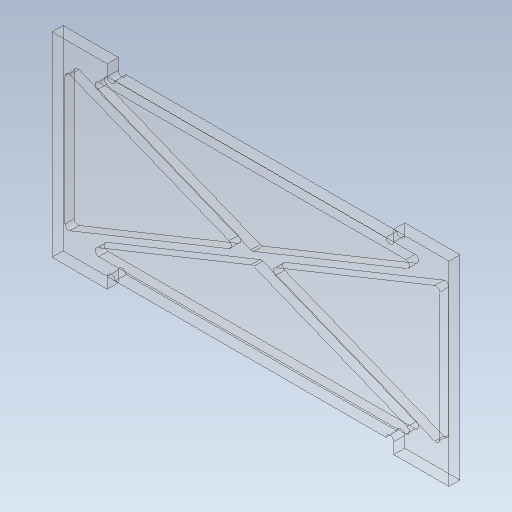
# Autodesk Inventor part: 台形サスバー板
Saved by Autodesk Inventor 2020 (Build 240168000, 168)
## iProperties
Created: 2019-09-18
Part Number: 台形サスバー板
Material: ポリカーボネート、クリア
Document SubType Name: Modeling
Designer: tanjihayato
Density: 1.2 g/cm^3
Appearance: ポリカーボネート - クリア
Mass: 18.8575 g
Surface Area: 114.914 cm^2
Volume: 15.7145 cm^3
Author: tanjihayato
Autodesk Inventor part; units mm, degrees
ref_plane "YZ Plane" through (0, 0, 0) normal (1, 0, 0) x (0, 1, 0)
ref_plane "XZ Plane" through (0, 0, 0) normal (0, 1, 0) x (-1, 0, 0)
ref_plane "XY Plane" through (0, 0, 0) normal (0, 0, 1) x (1, 0, 0)
sketch "スケッチ1" plane through (0, 0, 0) normal (0, 0, 1) x (1, 0, 0)
  circle A0 centre (-35.9404, 22.842) radius 1.5
  circle A1 centre (5.9362, 53.5882) radius 1.5
  circle A2 centre (127.6431, 30.2622) radius 1.5
  line L0 (22.1499, 50.4807) -> (113.9448, 32.8876)
  circle A3 centre (5.9362, 53.5882) radius 4.5
  circle A4 centre (127.6431, 30.2622) radius 4.5
  circle A5 centre (-35.9404, 22.842) radius 3
  line L1 (5.0892, 49.1686) -> (11.145, 48.008)
  line L2 (11.145, 48.008) -> (22.1499, 50.4807)
  line L3 (113.9448, 32.8876) -> (122.4523, 26.6751)
  line L4 (122.4523, 26.6751) -> (126.7961, 25.8426)
  line L5 (4.4419, 57.8328) -> (15.2047, 61.622)
  line L6 (-37.785, 25.2079) -> (3.1694, 57.1371)
  line L7 (3.5126, 49.7966) -> (-34.0959, 20.4761)
  line L8 (122.0018, 41.1536) -> (130.601, 33.6535)
  circle A6 centre (80.3181, 36.2778) radius 3
  circle A7 centre (80.3181, 36.2778) radius 4.5
  line L9 (128.2106, 34.7263) -> (80.8855, 40.7419)
  circle A8 centre (80.4743, 23.124) radius 1.5
  line L10 (120.4636, 35.711) -> (121.0283, 38.6574)
  line L11 (15.1864, 58.9428) -> (14.6217, 55.9964)
  circle A9 centre (66.9779, 42.9073) radius 1.5
  circle A10 centre (66.9779, 42.9073) radius 3
  line L12 (29.9182, 56.1193) -> (29.3535, 53.1729)
  arc A11 (17.2488, 58.5475) -> (15.1864, 58.9428) centre (16.2176, 58.7451) ccw
  arc A12 (29.9182, 56.1193) -> (27.8558, 56.5146) centre (28.887, 56.3169) ccw
  arc A13 (27.2911, 53.5682) -> (29.3535, 53.1729) centre (28.3223, 53.3705) ccw
  arc A14 (14.6217, 55.9964) -> (16.6841, 55.6011) centre (15.6529, 55.7987) ccw
  line L13 (17.2488, 58.5475) -> (27.8558, 56.5146)
  line L14 (16.6841, 55.6011) -> (27.2911, 53.5682)
  arc A15 (31.8825, 55.7428) -> (27.0019, 58.7146) centre (28.887, 56.3169) ccw
  line L15 (27.0019, 58.7146) -> (18.8556, 60.2759)
  arc A16 (18.8556, 60.2759) -> (15.2047, 61.622) centre (16.2176, 58.7451) ccw
  line L16 (106.2964, 41.4808) -> (105.7317, 38.5345)
  arc A17 (108.3589, 41.0856) -> (106.2964, 41.4808) centre (107.3276, 41.2832) ccw
  arc A18 (121.0283, 38.6574) -> (118.9658, 39.0527) centre (119.997, 38.855) ccw
  arc A19 (118.4011, 36.1063) -> (120.4636, 35.711) centre (119.4323, 35.9086) ccw
  arc A20 (105.7317, 38.5345) -> (107.7942, 38.1392) centre (106.7629, 38.3368) ccw
  line L17 (31.8825, 55.7428) -> (104.3322, 41.8573)
  line L18 (108.3589, 41.0856) -> (118.9658, 39.0527)
  line L19 (107.7942, 38.1392) -> (118.4011, 36.1063)
  arc A21 (122.0018, 41.1536) -> (118.1119, 41.2527) centre (119.997, 38.855) ccw
  line L20 (118.1119, 41.2527) -> (109.9656, 42.814)
  arc A22 (109.9656, 42.814) -> (104.3322, 41.8573) centre (107.3276, 41.2832) ccw
  line L21 (30.3885, 58.9717) -> (38.2584, 54.5208)
  line L22 (16.7917, 61.7406) -> (29.4611, 59.3124)
  line L23 (120.5711, 41.8505) -> (107.9017, 44.2787)
  line L24 (106.8479, 44.2952) -> (98.5267, 42.97)
  point P0 (0, 0)
  point P1 (0, 0)
  point P2 (0, 0)
  dimension "d53" = 9
  dimension "d49" = 9
  dimension "d50" = 9
  dimension "d51" = 6
  dimension "d52" = 6
  dimension "d54" = 47.7059
  dimension "d55" = 47.7059
  dimension "d56" = 3
  dimension "d57" = 3
  dimension "d58" = 8.0769
  dimension "d59" = 8.0769
  dimension "d60" = 3
  dimension "d61" = 6
  dimension "d62" = 61.9691
  dimension "d63" = 61.9691
  dimension "d64" = 15
  dimension "d65" = 2.1
  dimension "d66" = 2
  dimension "d67" = 2
  dimension "d68" = 2
  dimension "d69" = 15
  dimension "d70" = 2.1
  dimension "d71" = 7
  dimension "d72" = 2
  dimension "d73" = 2
  constraints: 50 end point, 39 point on circle, 26 tangent, 22 centre point, 13 point on line, 9 perpendicular, 7 parallel, 6 equal radius, 5 coincident, 2 collinear, 5 other
  measures "d49" diameter of A3
  measures "d50" diameter of A4
  measures "d51" diameter of A5
  measures "d52" diameter of A6
  measures "d54" distance of A8.centre A2.centre
  measures "d55" distance of A2.centre A6.centre
  measures "d56" distance of L10.start L10.end
  measures "d57" distance of L11.start L11.end
  measures "d58" distance from line of A2.centre L10
  measures "d59" distance from line of A1.centre L11
  measures "d60" diameter of A9
  measures "d61" diameter of A10
  measures "d62" distance of A2.centre A9.centre
  measures "d63" distance of A1.centre A9.centre
  measures "d64" distance of L12.start L11.start
  measures "d65" diameter of A11
  measures "d66" distance between parallel lines of L13 L15
  measures "d67" radial gap between concentric circles of A11 A16
  measures "d68" radial gap between concentric circles of A12 A15
  measures "d69" distance of L10.end L16.start
  measures "d70" diameter of A17
  measures "d71" distance between parallel lines of L0 L17
  measures "d72" distance between parallel lines of L18 L20
  measures "d73" radial gap between concentric circles of A21 A18
sketch "スケッチ2" plane through (0, 0, 0) normal (0, 0, 1) x (1, 0, 0)
  line L0 (17.1, 0) -> (90.6683, 0)
  line L1 (107.7683, 0) -> (107.7683, -47)
  line L2 (90.6683, -47) -> (17.1, -47)
  line L3 (0, -47) -> (0, 0)
  line L4 (0, 0) -> (0, 3)
  line L5 (0, 3) -> (15, 3)
  line L6 (15, 3) -> (15, 0)
  line L7 (107.7683, 0) -> (107.7683, 3)
  line L8 (107.7683, 3) -> (92.7683, 3)
  line L9 (92.7683, 3) -> (92.7683, 0)
  line L10 (107.7683, -47) -> (107.7683, -50)
  line L11 (107.7683, -50) -> (92.7683, -50)
  line L12 (92.7683, -50) -> (92.7683, -47)
  line L13 (0, -47) -> (0, -50)
  line L14 (0, -50) -> (15, -50)
  line L15 (15, -50) -> (15, -47)
  arc A0 (15, 0) -> (17.1, 0) centre (16.05, 0) ccw
  arc A1 (90.6683, 0) -> (92.7683, 0) centre (91.7183, 0) ccw
  arc A2 (92.7683, -47) -> (90.6683, -47) centre (91.7183, -47) ccw
  arc A3 (17.1, -47) -> (15, -47) centre (16.05, -47) ccw
  line L16 (15.1864, 58.9428) -> (14.6217, 55.9964) projected
  line L17 (120.4636, 35.711) -> (121.0283, 38.6574) projected
  dimension "d30" = 107.7683
  dimension "d31" = 47
  dimension "d32" = 3
  dimension "d33" = 15
  dimension "d34" = 3
  dimension "d35" = 15
  dimension "d36" = 3
  dimension "d37" = 15
  dimension "d38" = 3
  dimension "d39" = 3
  dimension "d40" = 15
  dimension "d41" = 2.1
  dimension "d42" = 2.1
  dimension "d43" = 2.1
  dimension "d44" = 2.1
  dimension "d45" = 3
  dimension "d46" = 3
  dimension "d74" = 107.7683
  constraints: 32 end point, 10 point on line, 8 point on circle, 7 perpendicular, 4 centre point, 4 tangent, 2 parallel, 2 vertical, 1 horizontal
  measures "d30" distance of L3.end L1.start
  measures "d31" distance between parallel lines of L2 L0
  measures "d32" distance of L3.end L4.end
  measures "d33" distance of L4.end L5.end
  measures "d34" distance of L1.start L7.end
  measures "d35" distance of L7.end L8.end
  measures "d36" distance of L1.end L10.end
  measures "d37" distance of L10.end L11.end
  measures "d38" distance of L12.end L11.end
  measures "d39" distance of L3.start L13.end
  measures "d40" distance of L13.end L14.end
  measures "d41" diameter of A0
  measures "d42" diameter of A1
  measures "d43" diameter of A2
  measures "d44" diameter of A3
  measures "d45" distance between parallel lines of L5 L0
  measures "d46" distance between parallel lines of L2 L14
  measures "d74" distance between parallel lines of L17 L16
extrude "押し出し1" add sketch "スケッチ2" along normal blind 3
sketch "スケッチ3" plane through (0, 0, 0) normal (0, 0, -1) x (-1, 0, 0)
  line L0 (0, 3) -> (0, -50) projected
  line L1 (-15, 3) -> (0, 3) projected
  line L2 (-15, 0) -> (-15, 3) projected
  arc A0 (-17.1, 0) -> (-15, 0) centre (-16.05, 0) ccw projected
  line L3 (-90.6683, 0) -> (-17.1, 0) projected
  arc A1 (-92.7683, 0) -> (-90.6683, 0) centre (-91.7183, 0) ccw projected
  line L4 (-92.7683, 3) -> (-92.7683, 0) projected
  line L5 (-107.7683, 3) -> (-92.7683, 3) projected
  line L6 (-107.7683, -50) -> (-107.7683, 3) projected
  line L7 (-92.7683, -50) -> (-107.7683, -50) projected
  line L8 (-92.7683, -47) -> (-92.7683, -50) projected
  arc A2 (-90.6683, -47) -> (-92.7683, -47) centre (-91.7183, -47) ccw projected
  line L9 (-17.1, -47) -> (-90.6683, -47) projected
  arc A3 (-15, -47) -> (-17.1, -47) centre (-16.05, -47) ccw projected
  line L10 (-15, -50) -> (-15, -47) projected
  line L11 (0, -50) -> (-15, -50) projected
  line L12 (-104.7683, -3) -> (-3, -3)
  line L13 (-3, -3) -> (-3, -44)
  line L14 (-3, -44) -> (-104.7683, -44)
  line L15 (-104.7683, -44) -> (-104.7683, -3)
  line L16 (-104.7683, -3) -> (-3, -44) construction
  arc A4 (-104.2078, -1.6087) -> (-106.2683, -3) centre (-104.7683, -3) ccw
  arc A5 (-3.5605, -45.3913) -> (-2.4395, -42.6087) centre (-3, -44) ccw
  line L17 (-3, -3) -> (-104.7683, -44) construction
  arc A6 (-2.4395, -4.3913) -> (-3.5605, -1.6087) centre (-3, -3) ccw
  arc A7 (-105.3288, -42.6087) -> (-104.2078, -45.3913) centre (-104.7683, -44) ccw
  line L18 (-3, -42.3828) -> (-49.8701, -23.5)
  line L19 (-53.8842, -21.8828) -> (-100.7543, -3)
  line L20 (-100.7543, -44) -> (-53.8842, -25.1172)
  line L21 (-49.8701, -23.5) -> (-3, -4.6172)
  line L22 (-104.7683, -4.6172) -> (-57.8982, -23.5)
  line L23 (-53.8842, -25.1172) -> (-7.014, -44)
  line L24 (-7.014, -3) -> (-53.8842, -21.8828)
  line L25 (-57.8982, -23.5) -> (-104.7683, -42.3828)
  point P0 (0, 0)
  point P1 (-53.8842, -23.5)
  point P2 (-53.8842, -23.5)
  dimension "d75" = 3
  dimension "d76" = 3
  dimension "d77" = 3
  dimension "d78" = 3
  dimension "d79" = 3
  dimension "d80" = 3
  constraints: 32 end point, 16 tangent, 10 parallel, 9 point on line, 8 point on circle, 4 centre point, 2 midpoint, 1 horizontal, 1 perpendicular
  measures "d75" distance between parallel lines of L12 L3
  measures "d76" distance between parallel lines of L14 L9
  measures "d77" distance between parallel lines of L0 L13
  measures "d78" distance between parallel lines of L6 L15
  measures "d79" diameter of A5
  measures "d80" diameter of A7
extrude "押し出し2" cut sketch "スケッチ3" against normal blind 2.5 contours L12 L24 L19 | L22 L25 L15 | L13 L18 L21 | L20 L23 L14
fillet "フィレット1" radius 1 12 edges at (100.7543, -3, 1.25) (104.7683, -4.6172, 1.25) (104.7683, -42.3828, 1.25) (100.7543, -44, 1.25) (57.8982, -23.5, 1.25) (53.8842, -21.8828, 1.25) (53.8842, -25.1172, 1.25) (49.8701, -23.5, 1.25) (7.014, -44, 1.25) (3, -42.3828, 1.25) (3, -4.6172, 1.25) (7.014, -3, 1.25)
equation "\"d55\" = d54"
equation "\"d59\" = d58"
equation "\"d63\" = d62"
equation "\"d30\" = d74"
